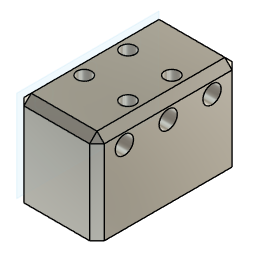
DASHBOARD_SUPPORT (Autodesk Fusion 360 design; units mm, degrees)
Autodesk Fusion 360 part; units mm, degrees
note: some values were not read from the file. Set by a fixed rule: which sketch regions a step uses.
sketch "Esquisse1" plane through (0, 0, 0) normal (0, 0, 1) x (1, 0, 0)
  line L0 (0, 0) -> (22, 0)
  line L1 (22, 0) -> (22, 39)
  line L2 (22, 39) -> (0, 39)
  line L3 (0, 39) -> (0, 0)
  circle A0 centre (5, 13.5) radius 2
  circle A1 centre (17, 13.5) radius 2
  circle A2 centre (5, 25.5) radius 2
  circle A3 centre (17, 25.5) radius 2
  dimension "d3" = 22
  dimension "d22" = 13.5
  dimension "d23" = 39
  dimension "d26" = 12
  dimension "d27" = 12
  constraint horizontal L0
  constraint vertical L1
  constraint horizontal L2
  constraint vertical L3
  constraint coincident L0.start L3.end
  measures "d3" distance of L0.start L0.end
  measures "d22" distance of L0 A0.centre
  measures "d23" distance of L0.start L2.end
extrude "Extrusion1" add sketch "Esquisse1" along normal blind 25
sketch "Esquisse2" plane through (22, 0, 0) normal (1, 0, 0) x (0, 1, 0)
  line L0 (0, 0) -> (39, 0)
  line L1 (39, 0) -> (39, 25)
  line L2 (39, 25) -> (0, 25)
  line L3 (0, 25) -> (0, 0)
  circle A0 centre (31.5, 20) radius 2.5
  circle A1 centre (19.5, 20) radius 2.5
  circle A2 centre (7.5, 20) radius 2.5
  dimension "d12" = 5
  dimension "d13" = 5
  dimension "d14" = 7.5
  dimension "d17" = -12
  dimension "d18" = 0
  measures "d12" diameter of A0
  measures "d13" distance of L2 A0.centre
  measures "d14" distance of L1 A0.centre
extrude "Extrusion2" cut sketch "Esquisse2" against normal blind 32 contours A0 | A1 | A2
sketch "Esquisse3" plane through (0, 0, 0) normal (-1, 0, 0) x (0, -1, 0)
  circle A0 centre (-31.5, 20) radius 2.5
  circle A1 centre (-19.5, 20) radius 2.5
  circle A2 centre (-7.5, 20) radius 2.5
  line L0 (-39, 0) -> (0, 0)
  line L1 (0, 0) -> (0, 25)
  line L2 (0, 25) -> (-39, 25)
  line L3 (-39, 25) -> (-39, 0)
chamfer "Chanfrein1" distance 2 angle 45 8 edges at (0, 0, 12.5) (22, 0, 12.5) (0, 19.5, 25) (22, 19.5, 25) (11, 0, 25) (11, 39, 25) (0, 39, 12.5) (22, 39, 12.5)
